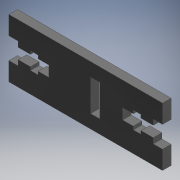
# Autodesk Inventor part: Part13
Saved by Autodesk Inventor 2019.2 (Build 232265000, 265)
## iProperties
Part Number: Part13
Material: Generic
Document SubType Name: Modeling
Designer: richard.girt
Mass: 2.23048 g
Surface Area: 22.232 cm^2
Volume: 2.23048 cm^3
Density: 1 g/cm^3
Appearance: Default
Author: richard.girt
Autodesk Inventor part; units mm, degrees
ref_plane "YZ Plane" through (0, 0, 0) normal (1, 0, 0) x (0, 1, 0)
ref_plane "XZ Plane" through (0, 0, 0) normal (0, 1, 0) x (-1, 0, 0)
ref_plane "XY Plane" through (0, 0, 0) normal (0, 0, 1) x (1, 0, 0)
sketch "Sketch1" plane through (0, 0, 0) normal (0, 0, 1) x (1, 0, 0)
  line L0 (25, 9.5) -> (-25, 9.5)
  line L1 (-25, 9.5) -> (-25, -9.5)
  line L2 (-25, -9.5) -> (25, -9.5)
  line L3 (25, -9.5) -> (25, 9.5)
  line L4 (25, 9.5) -> (-25, -9.5) construction
  line L5 (-25, 9.5) -> (25, -9.5) construction
  line L6 (4.6, 5.15) -> (1.6, 5.15)
  line L7 (1.6, 5.15) -> (1.6, -5.15)
  line L8 (1.6, -5.15) -> (4.6, -5.15)
  line L9 (4.6, -5.15) -> (4.6, 5.15)
  line L10 (4.6, 5.15) -> (1.6, -5.15) construction
  line L11 (1.6, 5.15) -> (4.6, -5.15) construction
  line L12 (-25, 3.5) -> (-22, 3.5)
  line L13 (-22, 3.5) -> (-22, -3.5)
  line L14 (-22, -3.5) -> (-25, -3.5)
  line L15 (-25, -3.5) -> (-25, 3.5)
  line L16 (-22, 1.75) -> (-12, 1.75)
  line L17 (-12, 1.75) -> (-12, -1.75)
  line L18 (-12, -1.75) -> (-22, -1.75)
  line L19 (-22, -1.75) -> (-22, 1.75)
  line L20 (-18, 2.8) -> (-15.5, 2.8)
  line L21 (-15.5, 2.8) -> (-15.5, -2.8)
  line L22 (-15.5, -2.8) -> (-18, -2.8)
  line L23 (-18, -2.8) -> (-18, 2.8)
  line L24 (0, 9.5) -> (0, -9.5) construction
  line L25 (25, 3.5) -> (22, 3.5)
  line L26 (22, 3.5) -> (22, -3.5)
  line L27 (22, -3.5) -> (25, -3.5)
  line L28 (25, -3.5) -> (25, 3.5)
  line L29 (22, 1.75) -> (12, 1.75)
  line L30 (12, 1.75) -> (12, -1.75)
  line L31 (12, -1.75) -> (22, -1.75)
  line L32 (22, -1.75) -> (22, 1.75)
  line L33 (18, 2.8) -> (15.5, 2.8)
  line L34 (15.5, 2.8) -> (15.5, -2.8)
  line L35 (15.5, -2.8) -> (18, -2.8)
  line L36 (18, -2.8) -> (18, 2.8)
  point P0 (0, 0)
  point P1 (3.1, 0)
  point P2 (0, 0)
  point P3 (3.1, 0)
  point P4 (-25, 0)
  point P5 (-22, 0)
  point P6 (-15.5, 0)
  point P7 (25, 0)
  point P8 (22, 0)
  point P9 (15.5, 0)
  dimension "d0" = 19
  dimension "d1" = 50
  dimension "d2" = 20.4
  dimension "d3" = 3
  dimension "d4" = 10.3
  dimension "d5" = 3
  dimension "d6" = 7
  dimension "d7" = 3.5
  dimension "d8" = 7
  dimension "d9" = 2.5
  dimension "d10" = 5.6
  dimension "d11" = 13
  constraints: 74 end point, 15 symmetric about line, 13 midpoint, 10 parallel, 5 horizontal, 5 perpendicular, 2 horizontal alignment, 2 point on line
  measures "d0" distance of L0.end L1.end
  measures "d1" distance of L0.start L0.end
  measures "d2" distance between parallel lines of L9 L3
  measures "d3" distance of L6.start L6.end
  measures "d4" distance of L8.end L6.start
  measures "d5" distance of L13.end L14.end
  measures "d6" distance between parallel lines of L12 L14
  measures "d7" distance of L16.end L17.end
  measures "d8" distance between parallel lines of L23 L1
  measures "d9" distance of L21.end L22.end
  measures "d10" distance of L20.end L21.end
  measures "d11" distance between parallel lines of L1 L17
extrude "Extrusion1" add sketch "Sketch1" along normal mid plane 2.8 contours L3 L25 L26 L29 L36 L33 L34 L30 L31 L35 L27 L2 L1 L14 L13 L18 L23 L22 L21 L17 L16 L20 L12 L0
body "Solid1"
